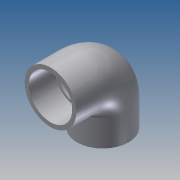
# Autodesk Inventor part: elbow_90deg_63mm
Saved by Autodesk Inventor 2014 SP1 (Build 180222100, 222)
## iProperties
Created: 2015-03-24
Part Number: elbow_90deg_63mm
Material: PVC-Piping
Document SubType Name: Modeling
Designer: Dave
Density: 1.4 g/cm^3
Appearance: Smooth - White
Mass: 301.746 g
Surface Area: 614.242 cm^2
Volume: 215.533 cm^3
Author: Dave
Autodesk Inventor part; units mm, degrees
ref_plane "YZ Plane" through (0, 0, 0) normal (1, 0, 0) x (0, 1, 0)
ref_plane "XY Plane" through (0, 0, 0) normal (0, 0, 1) x (1, 0, 0)
sketch "Sketch1" plane through (0, 0, 0) normal (0, 0, 1) x (1, 0, 0)
  circle A0 centre (0, 0) radius 31.5
  circle A1 centre (0, 0) radius 37.5
  dimension "d0" = 63
  dimension "d1" = 6
  constraints: 2 centre point, 1 coincident
  measures "d0" diameter of A0
  measures "d1" radial gap between concentric circles of A1 A0
extrude "Extrusion1" add sketch "Sketch1" along normal blind 38
ref_plane "Work Plane1" through (0, -38, 0) normal (0, 1, 0) x (-1, 0, 0)
sketch "Sketch3" plane through (0, -38, 0) normal (0, 1, 0) x (-1, 0, 0)
  circle A0 centre (0, -38) radius 37.5
  line L0 (-37.5, 0) -> (37.5, 0) projected
  circle A1 centre (0, -38) radius 31.5
  point P0 (0, 0)
  dimension "d5" = 75
  dimension "d6" = 38
  dimension "d7" = 6
  constraints: 2 centre point
  measures "d5" diameter of A0
  measures "d6" distance from line of A0.centre L0
  measures "d7" radial gap between concentric circles of A0 A1
extrude "Extrusion2" add sketch "Sketch3" against normal blind 38
sketch "Sketch5" plane through (0, 0, 0) normal (1, 0, 0) x (0, 1, 0)
  spline S0 degree 5 poles (0, 0) (-0.0001, -5.969) (-1.1716, -11.9382) (-3.517, -17.6) (-10.3014, -27.6986) (-20.4, -34.483) (-26.0618, -36.8284) (-32.031, -37.9999) (-38, -38) knots 0 0 0 0 0 0 0.5 0.5 0.5 1 1 1 1 1 1
  constraints: 3 other
sketch "Sketch6" plane through (0, 0, 0) normal (0, 0, -1) x (-1, 0, 0)
  circle A0 centre (0, 0) radius 37.5 projected
  circle A1 centre (0, 0) radius 28
  dimension "d13" = 56
  constraints: 1 centre point, 1 coincident
  measures "d13" diameter of A1
sweep "Sweep1" add profiles "Sketch6" path "Sketch5"
equation "curve S0 of \"Sketch5\": x = 38*cos(t) - 38; y = -1 mm * 38 ul * sin(1 deg * t); t from d11 to d12"
body "Solid1"
